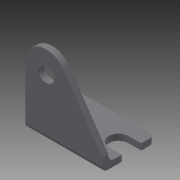
# Autodesk Inventor part: D-782_pin
Saved by Autodesk Inventor 2014 (Build 180170000, 170)
## iProperties
Created: 2014-01-19
Part Number: D-782_pin
Material: Steel
Catalog Web Link: www.cadenas.de
Description: Pivot Bracket for Original Line Cylinders - Right-
Vendor: BIMBA
Document SubType Name: Standard Catalog Part
Designer: Michael
Manufacturer: BIMBA
Density: 7.85 g/cm^3
Appearance: Steel
Mass: 5.11757 g
Surface Area: 10.1901 cm^2
Volume: 0.651919 cm^3
Category: PARTsolutions
Company: BIMBA
PSOL_IDENT_0: {$CADENAS_DATA\23d-libs\bimba\bimba\bimba_imperial\bimba_full_line\original_line_cylinders\accessori
PSOL_IDENT_1: es\pivot_bracket_right.prj},204 {VTYP=3D},{NB=D-782_pin},{LINA=D-782_pin},{NN=Pivot Bracket for Orig
PSOL_IDENT_2: inal Line Cylinders - Right},{DATE=06.12.2011 08:05:39},{GEOMDATE=06.12.2011 08:05:00},{VERSION=},{L
PSOL_IDENT_3: INEID=350},{LINESUBID=-1},{WBVAR=}  {NB=D-782_pin},{LINA=D-782_pin},{KT=DUMMY},{PN=D-782_pin},{MAT=Z
PSOL_IDENT_4: inc-Plated Carbon Steel},{CD=1},{L=0.75000000},{L1=0.50000000},{L2=0.25000000},{L3=0.37500000},{L5=0
PSOL_IDENT_5: .20300000},{L6=0.05980000},{H=0.77000000},{H1=0.12500000},{H2=0.56550000},{H22=0.5655},{W=0.51000000
PSOL_IDENT_6: },{W1=0.19000000},{W2=0.28350000},{R1=0.09500000},{R2=0.20300000},{R3=0.05000000},{D1=0.15850000},{C=
PSOL_IDENT_7: 1}
CNS_NN: Pivot Bracket for Original Line Cylinders - Right
CNS_NB: D-782_pin
CNS_NBSYN: $PN.
CNS_LINA: D-782_pin
CNS_PN: D-782_pin
CNS_MAT: Zinc-Plated Carbon Steel
CNS_CD: 1
CNS_L: 0.75000000
CNS_L1: 0.50000000
CNS_L2: 0.25000000
CNS_L3: 0.37500000
CNS_L5: 0.20300000
CNS_L6: 0.05980000
CNS_H: 0.77000000
CNS_H1: 0.12500000
CNS_H2: 0.56550000
CNS_H22: 0.566
CNS_W: 0.51000000
CNS_W1: 0.19000000
CNS_W2: 0.28350000
CNS_R1: 0.09500000
CNS_R2: 0.20300000
CNS_R3: 0.05000000
CNS_D1: 0.15850000
CNS_C: 1
SUPPLIER: BIMBA
ARTICLENO: D-782_pin
BOMINFO: D-782_pin
CREATOR: CADENAS GmbH
Title: D-782_pin
Author: Cadenas PARTsolutions
Autodesk Inventor part; units mm, degrees
sketch "Sketch_1" plane through (0, 0, 0) normal (1, 0, 0) x (0, 1, 0)
  line L0 (19.558, 0) -> (1.27, 0)
  arc A0 (1.27, 0) -> (0, -1.27) centre (1.27, -1.27) ccw
  line L1 (0, -1.27) -> (0, -12.954)
  line L2 (0, -12.954) -> (1.5189, -12.954)
  line L3 (1.5189, -12.954) -> (1.5189, -2.7889)
  arc A1 (2.7889, -1.5189) -> (1.5189, -2.7889) centre (2.7889, -2.7889) ccw
  line L4 (2.7889, -1.5189) -> (19.558, -1.5189)
  line L5 (19.558, -1.5189) -> (19.558, 0)
  constraints: 12 end point, 4 point on circle, 2 centre point
extrude "Extrusion1" add sketch "Sketch_1" along normal blind 19.05
sketch "Sketch_2" plane through (0, 0, 0) normal (0, 0, 1) x (1, 0, 0)
  line L0 (-19.05, -19.558) -> (28.575, -19.558)
  line L1 (28.575, -19.558) -> (28.575, 29.337)
  line L2 (28.575, 29.337) -> (-19.05, 29.337)
  line L3 (-19.05, 29.337) -> (-19.05, -19.558)
  line L4 (0, 0) -> (19.05, 0)
  line L5 (19.05, 0) -> (19.05, 3.175)
  line L6 (19.05, 3.175) -> (9.4129, 17.2734)
  arc A0 (9.4129, 17.2734) -> (0, 14.3637) centre (5.1562, 14.3637) ccw
  line L7 (0, 14.3637) -> (0, 0)
  constraints: 16 end point, 2 point on circle, 1 centre point
extrude "Extrusion2" cut sketch "Sketch_2" against normal blind 12.954
sketch "Sketch3" plane through (0, 1.27, 0) normal (0, 0, 1) x (1, 0, 0)
  point P0 (5.1562, 13.0937)
hole "Hole1" at (5.1562, 14.3637, 0) direction (0, 0, -1) diameter 4.0259 depth 1.5189
sketch "Sketch4" plane through (0, 0, -12.954) normal (0, -1, 0) x (1, 0, 0)
  point P0 (3.175, 5.7531)
hole "Hole2" at (3.175, 0, -7.2009) direction (0, 1, 0) diameter 4.826 depth 1.5189
sketch "Sketch5" plane through (0, 0, -12.954) normal (0, -1, 0) x (1, 0, 0)
  point P0 (15.875, 5.7531)
hole "Hole3" at (15.875, 0, -7.2009) direction (0, 1, 0) diameter 4.826 depth 1.5189
sketch "Sketch_6" plane through (0, 0, 0) normal (0, 1, 0) x (-1, 0, 0)
  line L0 (0, -9.6139) -> (0, -4.7879)
  line L1 (0, -4.7879) -> (-3.175, -4.7879)
  line L2 (-3.175, -4.7879) -> (-3.175, -9.6139)
  line L3 (-3.175, -9.6139) -> (0, -9.6139)
  constraints: 8 end point
sketch "Sketch_7" plane through (0, 0, 0) normal (0, 1, 0) x (-1, 0, 0)
  line L0 (-15.875, -9.6139) -> (-15.875, -4.7879)
  line L1 (-15.875, -4.7879) -> (-19.05, -4.7879)
  line L2 (-19.05, -4.7879) -> (-19.05, -9.6139)
  line L3 (-19.05, -9.6139) -> (-15.875, -9.6139)
  constraints: 8 end point
extrude "Extrusion3" cut sketch "Sketch_6" along normal blind 1.5189
extrude "Extrusion4" cut sketch "Sketch_7" along normal blind 1.5189
sketch "Sketch_8" plane through (0, 0, 0) normal (0, 1, 0) x (-1, 0, 0)
  line L0 (0, -19.431) -> (0, -11.684)
  arc A0 (-1.27, -12.954) -> (0, -11.684) centre (-1.27, -11.684) ccw
  line L1 (-1.27, -12.954) -> (-17.78, -12.954)
  arc A1 (-19.05, -11.684) -> (-17.78, -12.954) centre (-17.78, -11.684) ccw
  line L2 (-19.05, -11.684) -> (-19.05, -19.431)
  line L3 (-19.05, -19.431) -> (0, -19.431)
  constraints: 8 end point, 4 point on circle, 2 centre point
extrude "Extrusion5" cut sketch "Sketch_8" along normal blind 1.5189
ref_plane "c2_XY" through (0, 0, 0) normal (1, 0, 0) x (0, 0, -1)
ref_plane "c2_YZ" through (0, 0, 0) normal (0, 0, -1) x (0, 1, 0)
ref_plane "c2_ZX" through (0, 0, 0) normal (0, 1, 0) x (1, 0, 0)
ref_plane "k2_XY" through (0, 0, -12.954) normal (1, 0, 0) x (0, 0, -1)
ref_plane "k2_YZ" through (0, 0, -12.954) normal (0, 0, -1) x (0, 1, 0)
ref_plane "k2_ZX" through (0, 0, -12.954) normal (0, 1, 0) x (1, 0, 0)
ref_plane "to_dummy_R_XY" through (0, 0, 0) normal (0, 0, 1) x (1, 0, 0)
ref_plane "to_dummy_R_YZ" through (0, 0, 0) normal (1, 0, 0) x (0, 1, 0)
ref_plane "to_dummy_R_ZX" through (0, 0, 0) normal (0, 1, 0) x (0, 0, 1)
ref_plane "to_pin_R_XY" through (5.1562, 14.3637, 0) normal (0, 0, 1) x (1, 0, 0)
ref_plane "to_pin_R_YZ" through (5.1562, 14.3637, 0) normal (1, 0, 0) x (0, 1, 0)
ref_plane "to_pin_R_ZX" through (5.1562, 14.3637, 0) normal (0, 1, 0) x (0, 0, 1)
body "Solid1"
